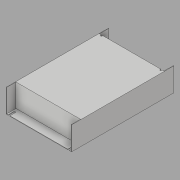
# Autodesk Inventor part: UHP-1500-230
Saved by Autodesk Inventor 2017 (Build 210142000, 142)
## iProperties
Created: 2022-09-19
Part Number: UHP-1500-230
Material: Generic
Document SubType Name: Modeling
Designer: JTS
Density: 1 g/cm^3
Appearance: Default
Author: JTS
Autodesk Inventor part; units mm, degrees
ref_plane "YZ Plane" through (0, 0, 0) normal (1, 0, 0) x (0, 1, 0)
ref_plane "XZ Plane" through (0, 0, 0) normal (0, 1, 0) x (-1, 0, 0)
sketch "Sketch1" plane through (0, 0, 0) normal (0, 0, 1) x (1, 0, 0)
  line L0 (-88.9, -31.75) -> (88.9, -31.75)
  line L1 (88.9, -31.75) -> (88.9, 31.75)
  line L2 (88.9, 31.75) -> (-88.9, 31.75)
  line L3 (-88.9, 31.75) -> (-88.9, -31.75)
  line L4 (-88.9, -31.75) -> (88.9, 31.75) construction
  line L5 (88.9, -31.75) -> (-88.9, 31.75) construction
  point P0 (0, 0)
  dimension "d0" = 177.8
  dimension "d1" = 63.5
  constraints: 12 end point, 2 horizontal, 2 midpoint, 2 vertical
  measures "d0" distance of L0.start L0.end
  measures "d1" distance of L2.end L0.start
extrude "Extrusion1" add sketch "Sketch1" along normal blind 278
sketch "Sketch2" plane through (-88.9, 31.75, 0) normal (0, 1, 0) x (1, 0, 0)
  line L0 (177.8, -278) -> (0, -278) projected
  line L1 (177.8, 0) -> (0, 0) projected
  arc A0 (10.15, -263.3) -> (5.65, -263.3) centre (7.9, -263.3) ccw
  arc A1 (172.15, -263.3) -> (167.65, -263.3) centre (169.9, -263.3) ccw
  arc A2 (167.65, -27) -> (172.15, -27) centre (169.9, -27) ccw
  arc A3 (5.65, -27) -> (10.15, -27) centre (7.9, -27) ccw
  line L2 (7.9, -263.3) -> (7.9, -27) construction
  line L3 (7.9, -27) -> (169.9, -27) construction
  line L4 (169.9, -27) -> (169.9, -263.3) construction
  line L5 (7.9, -27) -> (7.9, 0) construction
  line L6 (7.9, -27) -> (0, 0) construction
  line L7 (169.9, -27) -> (177.8, 0) construction
  line L8 (167.65, -263.3) -> (167.65, -278)
  line L9 (172.15, -263.3) -> (172.15, -278)
  line L10 (5.65, -263.3) -> (5.65, -278)
  line L11 (10.15, -263.3) -> (10.15, -278)
  line L12 (10.15, -27) -> (10.15, 0)
  line L13 (5.65, -27) -> (5.65, 0)
  line L14 (172.15, -27) -> (172.15, 0)
  line L15 (167.65, -27) -> (167.65, 0)
  point P0 (88.9, 0)
  dimension "d4" = 2.25
  dimension "d5" = 236.3
  dimension "d6" = 162
  dimension "d14" = 27
  constraints: 28 end point, 11 vertical, 9 point on line, 8 point on circle, 8 tangent, 4 centre point, 3 equal radius, 2 equal length, 1 coincident, 1 horizontal
  measures "d4" radius of A3
  measures "d5" distance of L2.start L2.end
  measures "d6" distance of L2.end L3.end
  measures "d14" distance of L2.end L5.end
extrude "Extrusion2" cut sketch "Sketch2" against normal up to surface (63.5 mm away)
ref_plane "Work Plane1" through (88.9, -30.48, 0) normal (0, -1, 0) x (1, 0, 0)
sketch "Sketch3" plane through (-88.9, 31.75, 278) normal (0, 1, 0) x (1, 0, 0)
  line L0 (0, 278) -> (0, 0) projected
  line L1 (177.8, 278) -> (177.8, 0) projected
  line L2 (176.53, 0) -> (176.53, 25.4)
  line L3 (176.53, 25.4) -> (1.27, 25.4)
  line L4 (1.27, 25.4) -> (1.27, 0)
  line L5 (1.27, 0) -> (176.53, 0)
  line L6 (1.27, 0) -> (0, 0) construction
  line L7 (177.8, 0) -> (176.53, 0) construction
  line L8 (1.27, 252.6) -> (176.53, 252.6)
  line L9 (176.53, 252.6) -> (176.53, 278)
  line L10 (176.53, 278) -> (1.27, 278)
  line L11 (1.27, 278) -> (1.27, 252.6)
  line L12 (1.27, 278) -> (0, 278) construction
  point P0 (88.9, 278)
  dimension "d9" = 1.27
  dimension "d10" = 25.4
  constraints: 22 end point, 6 horizontal, 4 collinear, 2 vertical
  measures "d9" distance of L4.end L0.end
  measures "d10" distance of L3.end L4.end
extrude "Extrusion3" cut sketch "Sketch3" against normal up to surface (62.23 mm away)
body "Solid1"
